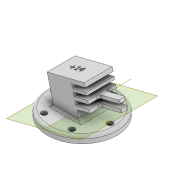
# Autodesk Inventor part: Plate_14
Saved by Autodesk Inventor 2022 (Build 260153000, 153)
## iProperties
Created: 2022-12-25
Part Number: Plate_14
Material: Generic
Document SubType Name: Modeling
Designer: dell
Density: 1 g/cm^3
Appearance: Default
Author: dell
Autodesk Inventor part; units mm, degrees
ref_plane "YZ Plane" through (0, 0, 0) normal (1, 0, 0) x (0, 1, 0)
ref_plane "XZ Plane" through (0, 0, 0) normal (0, 1, 0) x (-1, 0, 0)
ref_plane "XY Plane" through (0, 0, 0) normal (0, 0, 1) x (1, 0, 0)
sketch "Sketch1" plane through (0, 0, 0) normal (0, 1, 0) x (-1, 0, 0)
  circle A0 centre (0, 0) radius 50
  dimension "d0" = 100
  constraints: 1 centre point, 1 coincident
  measures "d0" diameter of A0
extrude "Extrusion1" add sketch "Sketch1" along normal blind 10
sketch "Sketch2" plane through (0, 10, 0) normal (0, 1, 0) x (1, 0, 0)
  circle A0 centre (-40, 0) radius 4.1
  point P0 (0, 0)
  dimension "d3" = 8.2
  dimension "d4" = 40
  constraints: 1 centre point
  measures "d3" diameter of A0
  measures "d4" distance of point (0, 0) A0.centre
extrude "Extrusion2" cut sketch "Sketch2" against normal blind 100
pattern_circular "Circular Pattern1" count 6 over 360 about axis through (0, 0, 0) along (0, 1, 0) of "Extrusion2"
ref_plane "Work Plane1" through (0, 10, -10) normal (0.2419219, -0.9702957, 0) x (0, 0, 1)
sketch "Sketch3" plane through (0, 10, 0) normal (-0.2419219, 0.9702957, 0) x (0.9702957, 0.2419219, 0)
  line L0 (-19.9192, 20) -> (15.0808, 20)
  line L1 (15.0808, 20) -> (15.0808, -20)
  line L2 (15.0808, -20) -> (-19.9192, -20)
  line L3 (-19.9192, -20) -> (-19.9192, 20)
  line L4 (-19.9192, 20) -> (15.0808, -20) construction
  line L5 (15.0808, 20) -> (-19.9192, -20) construction
  point P0 (-2.4192, 0)
  dimension "d10" = 35
  dimension "d11" = 40
  constraints: 12 end point, 2 midpoint, 2 parallel, 1 horizontal, 1 perpendicular
  measures "d10" distance of L1.end L2.end
  measures "d11" distance of L0.end L1.end
extrude "Extrusion3" add sketch "Sketch3" along normal blind 45
sketch "Sketch5" plane through (15.5425, 10, 20) normal (0.9702957, 0.2419219, 0) x (0, 0, -1)
  line L0 (0, 3.7601) -> (0, 48.7601) projected
  line L1 (40, 8.7265) -> (40, 48.7601) projected
  line L2 (0, 18.7601) -> (40, 18.7601)
  line L3 (40, 18.7601) -> (40, 13.7601)
  line L4 (40, 13.7601) -> (0, 13.7601)
  line L5 (0, 13.7601) -> (0, 18.7601)
  line L6 (0, 8.7265) -> (0, 48.7601) projected
  line L7 (0, 23.7601) -> (40, 23.7601)
  line L8 (40, 23.7601) -> (40, 28.7601)
  line L9 (40, 28.7601) -> (0, 28.7601)
  line L10 (0, 28.7601) -> (0, 23.7601)
  line L11 (40, 8.7265) -> (40, 48.7601) projected
  line L12 (0, 37.9601) -> (40, 37.9601)
  line L13 (40, 37.9601) -> (40, 33.7601)
  line L14 (40, 33.7601) -> (0, 33.7601)
  line L15 (0, 33.7601) -> (0, 37.9601)
  line L16 (0, 42.9601) -> (40, 42.9601)
  line L17 (40, 3.7601) -> (40, 48.7601) projected
  line L18 (0, 48.7601) -> (40, 48.7601) projected
  line L19 (0, 3.7601) -> (0, 48.7601) projected
  line L20 (0, 3.7601) -> (40, 3.7601) projected
  point P0 (20, -5.9429)
  point P1 (0, 0)
  point P2 (0, 13.7601)
  point P3 (0, 42.9601)
  point P4 (40, 42.9601)
  point P5 (0, 33.7601)
  point P6 (40, 33.7601)
  point P7 (40, 37.9601)
  point P8 (0, 37.9601)
  point P9 (0, 28.7601)
  point P10 (0, 23.7601)
  point P11 (40, 23.7601)
  dimension "d16" = 5
  dimension "d19" = 5
  dimension "d20" = 5
  dimension "d21" = 5
  dimension "d22" = 4.2
  dimension "d23" = 5
  dimension "d44" = 15
  constraints: 26 end point, 8 point on line, 6 parallel, 4 perpendicular, 3 horizontal
  measures "d16" distance between parallel lines of L2 L4
  measures "d19" distance between parallel lines of L7 L2
  measures "d20" distance between parallel lines of L7 L9
  measures "d21" distance between parallel lines of L9 L14
  measures "d22" distance between parallel lines of L14 L12
  measures "d23" distance between parallel lines of L12 L16
  measures "d44" distance between parallel lines of L20 L2
extrude "Extrusion4" add sketch "Sketch5" along normal blind 20 contours L0 L2 L1 L4 | L0 L9 L1 L7 | L0 L12 L1 L14 | L0 L18 L1 L16
sketch "Sketch7" plane through (34.9484, 14.8384, 20) normal (0.9702957, 0.2419219, 0) x (0, 0, -1)
  point P0 (20, -5.9429)
sketch "Sketch6" plane through (34.9484, 14.8384, 20) normal (0.9702957, 0.2419219, 0) x (0, 0, -1)
  line L0 (40, 13.7601) -> (40, 18.7601) projected
  line L1 (40, 18.7601) -> (0, 18.7601) projected
  line L2 (0, 18.7601) -> (0, 13.7601) projected
  line L3 (0, 13.7601) -> (40, 13.7601) projected
  line L4 (0, 28.7601) -> (0, 23.7601) projected
  line L5 (0, 23.7601) -> (40, 23.7601) projected
  line L6 (40, 23.7601) -> (40, 28.7601) projected
  line L7 (40, 28.7601) -> (0, 28.7601) projected
  line L8 (40, 28.7601) -> (0, 28.7601) projected
  line L9 (15.5, 28.7601) -> (24.5, 28.7601)
  line L10 (24.5, 28.7601) -> (24.5, 23.7601)
  line L11 (24.5, 23.7601) -> (15.5, 23.7601)
  line L12 (15.5, 23.7601) -> (15.5, 28.7601)
  line L13 (40, 18.7601) -> (0, 18.7601) projected
  line L14 (15.5, 18.7601) -> (24.5, 18.7601)
  line L15 (24.5, 18.7601) -> (24.5, 13.7601)
  line L16 (24.5, 13.7601) -> (15.5, 13.7601)
  line L17 (15.5, 13.7601) -> (15.5, 18.7601)
  line L18 (20, -34.9382) -> (20, 83.3564) projected
  point P0 (20, -5.9429)
  point P1 (24.5, 18.7601)
  point P2 (15.5, 18.7601)
  point P3 (15.5, 13.7601)
  point P4 (24.5, 28.7601)
  dimension "d24" = 9
  dimension "d25" = 9
  dimension "d26" = 4.5
  dimension "d27" = 4.5
  constraints: 16 end point, 4 parallel, 4 point on line, 2 horizontal, 2 perpendicular
  measures "d24" distance between parallel lines of L10 L12
  measures "d25" distance between parallel lines of L17 L15
  measures "d26" distance between parallel lines of L18 L12
  measures "d27" distance between parallel lines of L18 L17
extrude "Extrusion5" add sketch "Sketch6" along normal blind 30 contours L3 L18 L1 L15 | L3 L17 L1 L18 | L7 L18 L5 L12 | L7 L10 L5 L18
thicken "Thicken1" operation add thickness 0.2 both sides no extend neighbours yes toward (0.2419219, -0.9702957, 0) faces at (17.4726, 29.8156, 1.5)
thicken "Thicken2" operation add thickness 0.2 both sides no extend neighbours yes toward (-0.2419219, 0.9702957, 0) faces at (16.263, 34.6671, -1.5)
thicken "Thicken3" operation add thickness 0.2 both sides no extend neighbours yes toward (0.2419219, -0.9702957, 0) faces at (15.0534, 39.5186, -1.5)
thicken "Thicken4" operation add thickness 0.2 both sides no extend neighbours yes toward (-0.2419219, 0.9702957, 0) faces at (13.8438, 44.3701, 6.6667)
thicken "Thicken5" operation add thickness 0.2 both sides no extend neighbours yes toward (0.2419219, -0.9702957, 0) faces at (19.2964, 50.0581, 6.6667)
thicken "Thicken6" operation add thickness 0.2 both sides no extend neighbours yes toward (-0.2419219, 0.9702957, 0) faces at (11.6181, 53.2968, 6.6667)
fillet "Fillet1" radius 3 8 edges at (-20.529, 10, 0) (-10.2645, 10, -20) (-10.2645, 10, 20) (12.2136, 23.3513, 0) (31.0389, 30.5185, -4.5) (28.5955, 40.3185, -4.5) (28.5955, 40.3185, 4.5) (31.0389, 30.5185, 4.5)
chamfer "Chamfer1" distance 14 angle 45 3 edges at (0, 10, -21.5) (0, 10, 0) (0, 10, 21.5)
fillet "Fillet3" radius 10 3 edges at (14, 10, 0) (14, 10, 21.5) (14, 10, -21.5)
fillet "Fillet4" radius 4 1 edges at (50, 10, 0)
sketch "Sketch8" plane through (-10.8865, 53.6633, 0) normal (-0.2419219, 0.9702957, 0) x (0.9702957, 0.2419219, 0)
  line L0 (-6.9685, 4.6888) -> (10.8183, 4.6888) construction
  line L1 (10.8183, 4.6888) -> (10.8183, -13.2224) construction
  line L2 (10.8183, -13.2224) -> (-6.9685, -13.2224) construction
  line L3 (-6.9685, -13.2224) -> (-6.9685, 4.6888) construction
  line L4 (0.1952, -0.2642) -> (-2.5147, -0.2642)
  line L5 (-2.5147, -0.2642) -> (-2.5147, -2.9741)
  line L6 (-2.5147, -2.9741) -> (-3.4093, -2.9741)
  line L7 (-3.4093, -2.9741) -> (-3.4093, -0.2642)
  line L8 (-3.4093, -0.2642) -> (-6.1192, -0.2642)
  line L9 (-6.1192, -0.2642) -> (-6.1192, 0.598)
  line L10 (-6.1192, 0.598) -> (-3.4093, 0.598)
  line L11 (-3.4093, 0.598) -> (-3.4093, 3.3079)
  line L12 (-3.4093, 3.3079) -> (-2.5147, 3.3079)
  line L13 (-2.5147, 3.3079) -> (-2.5147, 0.598)
  line L14 (-2.5147, 0.598) -> (0.1952, 0.598)
  line L15 (0.1952, 0.598) -> (0.1952, -0.2642)
  line L16 (6.1531, -3.3372) -> (2.2503, -3.3372)
  line L17 (2.2503, -3.3372) -> (2.2503, -2.5203)
  line L18 (2.2503, -2.5203) -> (3.7025, -2.5203)
  line L19 (3.7025, -2.5203) -> (3.7025, 2.8411)
  line L20 (3.7025, 2.8411) -> (2.2503, 2.8411)
  line L21 (2.2503, 2.8411) -> (2.2503, 3.5737)
  spline S0 degree 2 poles (2.2503, 3.5737) (3.0736, 3.5737) (3.8516, 4.0405) (3.9035, 4.6888) knots 0 0 0 1 2 2 2
  line L22 (3.9035, 4.6888) -> (4.7333, 4.6888)
  line L23 (4.7333, 4.6888) -> (4.7333, -2.5203)
  line L24 (4.7333, -2.5203) -> (6.1531, -2.5203)
  line L25 (6.1531, -2.5203) -> (6.1531, -3.3372)
  line L26 (12.7722, -0.5884) -> (11.8192, -0.5884)
  line L27 (11.8192, -0.5884) -> (11.8192, -3.3372)
  line L28 (11.8192, -3.3372) -> (10.7884, -3.3372)
  line L29 (10.7884, -3.3372) -> (10.7884, -0.5884)
  line L30 (10.7884, -0.5884) -> (7.2552, -0.5884)
  line L31 (7.2552, -0.5884) -> (7.2552, 0.5397)
  line L32 (7.2552, 0.5397) -> (10.8338, 4.6628)
  line L33 (10.8338, 4.6628) -> (11.8192, 4.6628)
  line L34 (11.8192, 4.6628) -> (11.8192, 0.2739)
  line L35 (11.8192, 0.2739) -> (12.7722, 0.2739)
  line L36 (12.7722, 0.2739) -> (12.7722, -0.5884)
  line L37 (10.7884, 0.2739) -> (10.7884, 3.3987)
  line L38 (10.7884, 3.3987) -> (8.098, 0.2739)
  line L39 (8.098, 0.2739) -> (10.7884, 0.2739)
  point P0 (-2.4192, 0)
  constraints: 2 other
extrude "Extrusion6" cut sketch "Sketch8" against normal blind 1
fillet "Fillet5" radius 1 4 edges at (60.1478, 37.7761, 4.5) (57.7044, 47.5761, 4.5) (57.7044, 47.5761, -4.5) (60.1478, 37.7761, -4.5)
equation "\"d26\" = 0.5 * d24"
equation "\"d27\" = 0.5 * d25"
body "Solid1"
